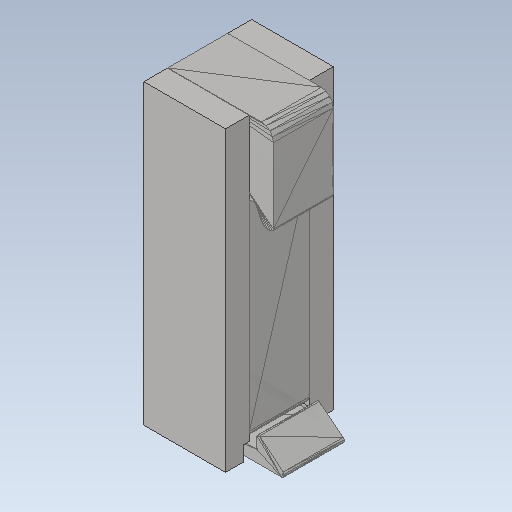
# Autodesk Inventor part: DIN_mount
Saved by Autodesk Inventor 2021 (Build 250183000, 183)
## iProperties
Created: 2020-05-12
Part Number: DIN_mount
Material: Generic
Document SubType Name: Modeling
Designer: Mateusz
Density: 1 g/cm^3
Appearance: Default
Author: Mateusz
Autodesk Inventor part; units mm, degrees
ref_plane "YZ Plane" through (0, 0, 0) normal (1, 0, 0) x (0, 1, 0)
ref_plane "XZ Plane" through (0, 0, 0) normal (0, 1, 0) x (-1, 0, 0)
ref_plane "XY Plane" through (0, 0, 0) normal (0, 0, 1) x (1, 0, 0)
sketch "Sketch1" plane through (13.782, 4.103, 5) normal (0, 0, 1) x (1, 0, 0)
  line L0 (-13.641, 45.75) -> (-13.641, -3.962) projected
  line L1 (2, 45.75) -> (-13.641, 45.75) projected
  line L2 (-13.641, -3.962) -> (-13.641, 45.75)
  line L3 (-13.641, 45.75) -> (0, 45.75)
  line L4 (0, 45.75) -> (0, 33.5)
  line L5 (0, 33.5) -> (0, -3.962)
  line L6 (0, -3.962) -> (-13.641, -3.962)
  point P0 (-13.782, -4.103)
  constraints: 10 end point, 2 point on line, 2 vertical, 1 perpendicular
extrude "Extrusion1" add sketch "Sketch1" along normal blind 4
sketch "Sketch2" plane through (4.5, 3.103, -5) normal (0, 0, -1) x (-1, 0, 0)
  line L0 (4.359, 46.75) -> (4.359, -2.962) projected
  line L1 (4.359, -2.962) -> (4.359, 46.75)
  line L2 (-9.282, 46.75) -> (4.359, 46.75) projected
  line L3 (4.359, 46.75) -> (-9.282, 46.75)
  line L4 (4.359, -2.962) -> (-9.282, -2.962) projected
  line L5 (-9.282, 46.75) -> (-9.282, -2.962)
  line L6 (-9.282, -2.962) -> (4.359, -2.962)
  point P0 (4.5, -3.103)
  constraints: 8 end point, 2 collinear, 2 perpendicular
extrude "Extrusion2" add sketch "Sketch2" along normal blind 4
sketch "Sketch3" plane through (0.141, 0.141, 5) normal (0, -1, 0) x (1, 0, 0)
  line L0 (0, 0) -> (13.641, 0) projected
  line L1 (13.641, 0) -> (13.641, 1)
  line L2 (13.641, 0) -> (13.641, 4) projected
  line L3 (13.641, 1) -> (0, 1)
  line L4 (0, 0) -> (0, 4) projected
  line L5 (0, 1) -> (0, 0)
  line L6 (0, 0) -> (13.641, 0)
  line L7 (0, -10) -> (13.641, -10) projected
  line L8 (13.641, -10) -> (13.641, -11)
  line L9 (13.641, -10) -> (13.641, -14) projected
  line L10 (13.641, -11) -> (0, -11)
  line L11 (0, -10) -> (0, -14) projected
  line L12 (0, -10) -> (0, -11)
  line L13 (0, -10) -> (13.641, -10)
  point P0 (-0.141, -5)
  dimension "d4" = 1
  dimension "d5" = 1
  constraints: 16 end point, 5 perpendicular, 4 point on line, 1 vertical
  measures "d4" distance of L0.end L1.end
  measures "d5" distance of L7.end L8.end
extrude "Extrusion3" cut sketch "Sketch3" against normal blind 2.5
body "Solid1"
